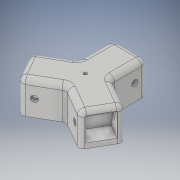
# Autodesk Inventor part: 80_20_top_connector
Saved by Autodesk Inventor 2019.4 (Build 234330000, 330)
## iProperties
Created: 2020-01-31
Part Number: 80_20_top_connector
Material: Generic
Document SubType Name: Modeling
Designer: Jorian Bruslind
Density: 1 g/cm^3
Appearance: Default
Author: Jorian Bruslind
Autodesk Inventor part; units mm, degrees
ref_plane "YZ Plane" through (0, 0, 0) normal (1, 0, 0) x (0, 1, 0)
ref_plane "XZ Plane" through (0, 0, 0) normal (0, 1, 0) x (-1, 0, 0)
ref_plane "XY Plane" through (0, 0, 0) normal (0, 0, 1) x (1, 0, 0)
sketch "Sketch1" plane through (0, 0, 0) normal (0, 1, 0) x (-1, 0, 0)
  line L0 (0, 0) -> (30, 0)
  line L1 (30, 0) -> (30, -40)
  line L2 (30, -40) -> (0, -40)
  line L3 (0, -40) -> (0, 0)
  dimension "d0" = 30
  dimension "d1" = 40
  constraints: 8 end point, 2 parallel, 1 horizontal, 1 perpendicular
  measures "d0" distance of L1.end L2.end
  measures "d1" distance of L0.end L1.end
extrude "Extrusion1" add sketch "Sketch1" along normal blind 30
sketch "Sketch6" plane through (0, 30, 0) normal (0, 1, 0) x (1, 0, 0)
  line L0 (0, 0) -> (-15, 0)
  line L1 (-30, 0) -> (0, 0) projected
  circle A0 centre (-15, 0) radius 1.5
  dimension "d32" = 3
  constraints: 2 end point, 1 centre point, 1 coincident, 1 midpoint
  measures "d32" diameter of A0
extrude "Extrusion6" cut sketch "Sketch6" against normal blind 30
pattern_circular "Circular Pattern4" count 3 over 360 about axis through (-15, 30, 0) along (0, -1, 0) of "Extrusion1", "Extrusion6"
sketch "Sketch7" plane through (0, 0, -40) normal (0, 0, -1) x (-1, 0, 0)
  line L0 (4.5, 4.5) -> (25.5, 4.5)
  line L1 (25.5, 4.5) -> (25.5, 25.5)
  line L2 (25.5, 25.5) -> (4.5, 25.5)
  line L3 (4.5, 25.5) -> (4.5, 4.5)
  line L4 (15, 30) -> (15, 0) projected
  line L5 (4.5, 4.5) -> (25.5, 25.5) construction
  line L6 (25.5, 4.5) -> (4.5, 25.5) construction
  point P0 (0, 0)
  point P1 (15, 15)
  dimension "d38" = 21
  dimension "d39" = 21
  constraints: 12 end point, 3 midpoint, 2 parallel, 1 horizontal, 1 perpendicular
  measures "d38" distance of L2.end L1.end
  measures "d39" distance of L1.end L0.end
extrude "Extrusion7" cut sketch "Sketch7" against normal blind 15
pattern_circular "Circular Pattern5" count 3 over 360 about axis through (-15, 30, 0) along (0, -1, 0) of "Extrusion7"
sketch "Sketch8" plane through (-15, 0, 17.3205) normal (-0.5, 0, 0.8660254) x (0.8660254, 0, 0.5)
  line L0 (31.3397, 0) -> (31.3397, 30) projected
  line L1 (31.3397, 15) -> (21.3397, 15)
  circle A0 centre (21.3397, 15) radius 2.75
  point P0 (4.3301, 0)
  dimension "d45" = 10
  dimension "d46" = 5.5
  constraints: 2 end point, 1 centre point, 1 coincident, 1 horizontal, 1 midpoint
  measures "d45" distance of L1.start L1.end
  measures "d46" diameter of A0
extrude "Extrusion8" cut sketch "Sketch8" against normal blind 30
pattern_circular "Circular Pattern6" count 3 over 360 about axis through (-15, 30, 0) along (0, -1, 0) of "Extrusion8"
fillet "Fillet5" radius 5 3 edges at (-15, 15, 17.3205) (0, 15, -8.6603) (-30, 15, -8.6603)
fillet "Fillet6" radius 5 9 edges at (-30, 30, -25.7735) (-44.8205, 30, -0.1036) (-30.6699, 30, -9.047) (-15, 30, 18.094) (-0.1795, 30, 25.8771) (-29.8205, 30, 25.8771) (0.6699, 30, -9.047) (14.8205, 30, -0.1036) (0, 30, -25.7735)
fillet "Fillet7" radius 4 15 edges at (-28.5355, 28.5355, -40) (-30, 12.5, -40) (-1.4645, 28.5355, -40) (0, 12.5, -40) (-15, 30, -40) (-42.8732, 28.5355, 31.7221) (-42.141, 12.5, 32.9904) (-56.4088, 28.5355, 8.2779) (-57.141, 12.5, 7.0096) (-49.641, 30, 20) (26.4088, 28.5355, 8.2779) (27.141, 12.5, 7.0096) (12.8732, 28.5355, 31.7221) (12.141, 12.5, 32.9904) (19.641, 30, 20)
body "Solid1"
